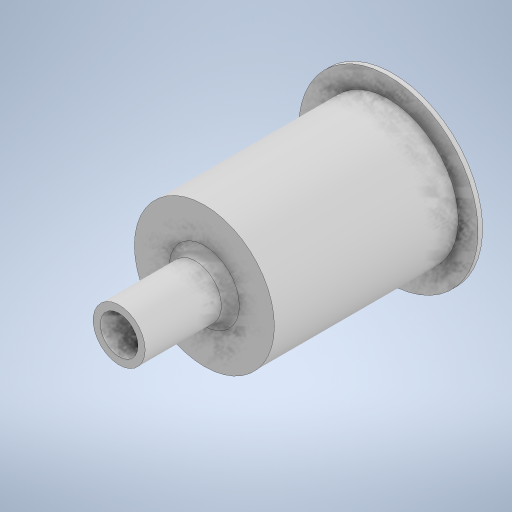
# Autodesk Inventor part: Smoke connector
Saved by Autodesk Inventor 2023 (Build 270158000, 158)
## iProperties
Created: 2022-10-05
Part Number: Smoke connector
Material: Generic
Document SubType Name: Modeling
Designer: earls
Density: 1 g/cm^3
Appearance: Default
Mass: 77.3696 g
Surface Area: 630.58 cm^2
Volume: 77.3696 cm^3
Author: earls
## iProperties of the stored document Smoke connector_3DPrint.ipt
Created: 2022-10-18
Part Number: Smoke connector_3DPrint
Material: Generic
Document SubType Name: Modeling
Designer: earls
Density: 1 g/cm^3
Appearance: Default
Author: earls
Autodesk Inventor part; units mm, degrees
ref_plane "YZ Plane" through (0, 0, 0) normal (1, 0, 0) x (0, 1, 0)
ref_plane "XZ Plane" through (0, 0, 0) normal (0, 1, 0) x (-1, 0, 0)
ref_plane "XY Plane" through (0, 0, 0) normal (0, 0, 1) x (1, 0, 0)
sketch "Sketch1" plane through (0, 0, 0) normal (0, 0, 1) x (1, 0, 0)
  circle A0 centre (0, 0) radius 39
  circle A1 centre (0, 0) radius 35
  dimension "d0" = 78
  dimension "d1" = 4
  constraints: 2 centre point, 1 coincident
  measures "d0" diameter of A0
  measures "d1" radial gap between concentric circles of A0 A1
extrude "Extrusion1" add sketch "Sketch1" along normal blind 100
sketch "Sketch2" plane through (0, 0, 100) normal (0, 0, 1) x (1, 0, 0)
  circle A0 centre (0, 0) radius 35 projected
  circle A1 centre (0, 0) radius 10.5
  circle A2 centre (0, 0) radius 14.5
  dimension "d4" = 21
  dimension "d5" = 4
  constraints: 2 centre point, 1 coincident
  measures "d4" diameter of A1
  measures "d5" radial gap between concentric circles of A1 A2
extrude "Extrusion2" add sketch "Sketch2" against normal blind 2.5 contours A0
extrude "Extrusion3" add sketch "Sketch2" along normal blind 50 contours A2
sketch "Sketch3" plane through (0, 0, 0) normal (0, 0, -1) x (-1, 0, 0)
  circle A0 centre (0, 0) radius 39 projected
  circle A1 centre (0, 0) radius 35 projected
  circle A2 centre (0, 0) radius 50
  dimension "d10" = 100
  constraints: 1 centre point, 1 coincident
  measures "d10" diameter of A2
extrude "Extrusion4" add sketch "Sketch3" along normal blind 2.5 contours A0 | A2
sketch "Sketch4" plane through (0, 0, 100) normal (0, 0, 1) x (1, 0, 0)
  circle A0 centre (0, 0) radius 14.5 projected
  circle A1 centre (0, 0) radius 39 projected
  circle A2 centre (0, 0) radius 14.5 projected
extrude "Extrusion5" add sketch "Sketch4" along normal blind 2.5
fillet "Fillet1" radius 5 1 edges at (-14.5, 0, 102.5)
fillet "Fillet2" radius 5 1 edges at (-14.5, 0, 100)
body "Solid1"
